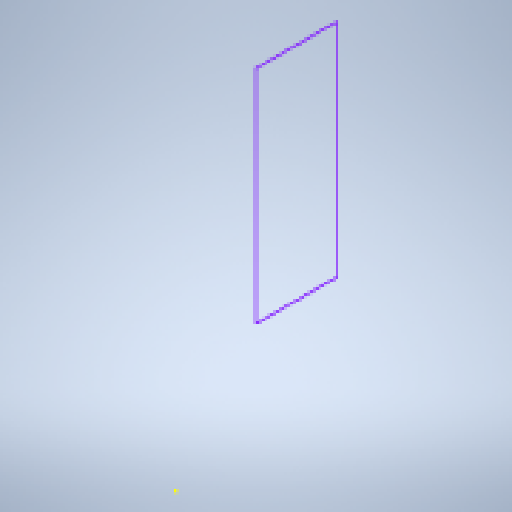
# Autodesk Inventor part: grabber arm
Saved by Autodesk Inventor 2023 (Build 270158000, 158)
## iProperties
Created: 2022-09-11
Part Number: grabber arm
Material: Generic
Document SubType Name: Modeling
Designer: deli
Density: 1 g/cm^3
Appearance: Default
Author: deli
Autodesk Inventor part; units mm, degrees
ref_plane "YZ Plane" through (0, 0, 0) normal (1, 0, 0) x (0, 1, 0)
ref_plane "XZ Plane" through (0, 0, 0) normal (0, 1, 0) x (-1, 0, 0)
ref_plane "XY Plane" through (0, 0, 0) normal (0, 0, 1) x (1, 0, 0)
sketch "Sketch1" plane through (0, 0, 0) normal (1, 0, 0) x (0, 1, 0)
  arc A0 (235.6561, 11.9476) -> (233.4201, 12.1711) centre (234.3735, 10.413) ccw projected
  line L0 (233.4201, 12.1711) -> (233.0465, 12.1697) projected
  arc A1 (233.0465, 12.1697) -> (233.6477, 14.6124) centre (226.9075, 14.9759) ccw projected
  arc A2 (233.6477, 14.6124) -> (231.9484, 16.6978) centre (231.6506, 14.7201) ccw projected
  arc A3 (228.5928, 20.0291) -> (231.9484, 16.6978) centre (232.5439, 20.6532) ccw projected
  arc A4 (228.5928, 20.0291) -> (226.4952, 21.7133) centre (226.6173, 19.7171) ccw projected
  arc A5 (226.4952, 21.7133) -> (223.3459, 20.7098) centre (226.9075, 14.9759) ccw projected
  arc A6 (223.3459, 20.7098) -> (223.8159, 23.7024) centre (222.2906, 22.4088) ccw projected
  arc A7 (229.6848, 29.1282) -> (223.8159, 23.7024) centre (226.8666, 26.2896) ccw construction
  line L1 (229.6848, 29.1282) -> (241.0393, 17.8555) projected
  arc A8 (235.6561, 11.9476) -> (241.0393, 17.8555) centre (238.2211, 15.0169) ccw projected
  arc A9 (228.735, 27.003) -> (227.7127, 28.1018) centre (226.8666, 26.2896) ccw construction
  arc A10 (227.7127, 28.1018) -> (228.735, 27.003) centre (226.8666, 26.2896) ccw construction
  arc A11 (230.6873, 21.3969) -> (231.7273, 22.4789) centre (232.5439, 20.6532) ccw construction
  arc A12 (231.7273, 22.4789) -> (230.6873, 21.3969) centre (232.5439, 20.6532) ccw construction
  arc A13 (238.9346, 13.1485) -> (240.0334, 14.1708) centre (238.2211, 15.0169) ccw construction
  arc A14 (240.0334, 14.1708) -> (238.9346, 13.1485) centre (238.2211, 15.0169) ccw construction
  arc A15 (234.2218, 14.9471) -> (241.0393, 17.8555) centre (238.2211, 15.0169) ccw
  arc A16 (228.8014, 20.4163) -> (232.334, 16.9091) centre (232.5439, 20.6532) ccw
  arc A17 (234.2218, 14.9471) -> (232.334, 16.9091) centre (232.2221, 14.9122) ccw
  arc A18 (228.8014, 20.4163) -> (226.8258, 22.2898) centre (226.8054, 20.2899) ccw
  arc A19 (223.8159, 23.7024) -> (226.8258, 22.2898) centre (226.8666, 26.2896) ccw
  line L2 (241.0393, 17.8555) -> (189.9876, 68.5392)
  line L3 (224.0484, 23.4509) -> (189.9596, 57.294)
  arc A20 (189.9876, 68.5392) -> (183.9717, 68.1036) centre (187.1694, 65.7005) ccw
  circle A21 centre (238.2211, 15.0169) radius 2
  circle A22 centre (232.5439, 20.6532) radius 2
  circle A23 centre (226.8258, 26.2485) radius 2
  circle A24 centre (187.1694, 65.7005) radius 2
  line L4 (183.9717, 68.1036) -> (172.9274, 57.4077)
  arc A25 (172.9274, 57.4077) -> (178.4896, 51.6577) centre (175.7101, 54.5343) ccw
  line L5 (184.362, 57.3319) -> (178.4896, 51.6577)
  arc A26 (189.9596, 57.294) -> (184.362, 57.3319) centre (187.1415, 54.4553) ccw
  circle A27 centre (175.7101, 54.5343) radius 2
  point P0 (0, 0)
  point P1 (235.6561, 11.9476)
  point P2 (223.8941, 23.6041)
  point P3 (241.0393, 17.8555)
  point P4 (235.6561, 11.9476)
  dimension "d0" = 7.5
  dimension "d1" = 4
  dimension "d2" = 4
  dimension "d3" = 8
  dimension "d4" = 8
  dimension "d6" = 8
  dimension "d7" = 60
  dimension "d8" = 4
  dimension "d9" = 4
  dimension "d10" = 4
  dimension "d13" = 4
  dimension "d17" = 8
  dimension "d18" = 8
  dimension "d19" = 4
  dimension "d20" = 16
  constraints: 18 point on circle, 13 centre point, 11 tangent, 9 end point, 6 coincident, 2 concentric, 1 parallel, 1 point on line
  measures "d0" diameter of A16
  measures "d1" diameter of A17
  measures "d2" diameter of A18
  measures "d3" diameter of A19
  measures "d4" diameter of A15
  measures "d6" diameter of A20
  measures "d7" distance of L3.start L4.start
  measures "d8" diameter of A21
  measures "d9" diameter of A23
  measures "d10" diameter of A22
  measures "d13" diameter of A24
  measures "d17" diameter of A25
  measures "d18" diameter of A26
  measures "d19" diameter of A27
  measures "d20" distance of A27.centre A24.centre
extrude "Extrusion1" add sketch "Sketch1" along normal blind 3.175
equation "\"d2\" = d1"
equation "\"d3\" = d4"
equation "\"d6\" = d3"
equation "\"d9\" = d8"
equation "\"d10\" = d8"
body "Solid1"
